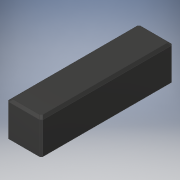
# Autodesk Inventor part: 1-Battery-Case
Saved by Autodesk Inventor 2019 (Build 230136000, 136)
## iProperties
Created: 2018-11-25
Part Number: 1-Battery-Case
Material: Generic
Document SubType Name: Modeling
Designer: lateSWE
Density: 1 g/cm^3
Appearance: Default
Author: lateSWE
Autodesk Inventor part; units mm, degrees
ref_plane "YZ Plane" through (0, 0, 0) normal (1, 0, 0) x (0, 1, 0)
ref_plane "XZ Plane" through (0, 0, 0) normal (0, 1, 0) x (-1, 0, 0)
ref_plane "XY Plane" through (0, 0, 0) normal (0, 0, 1) x (1, 0, 0)
sketch "Sketch1" plane through (0, 0, 0) normal (0, 0, 1) x (1, 0, 0)
  line L0 (0, 0) -> (22.5, 0)
  line L1 (22.5, 0) -> (22.5, 22.5)
  line L2 (22.5, 22.5) -> (0, 22.5)
  line L3 (0, 22.5) -> (0, 0)
  line L4 (0, 0) -> (20.5, 0)
  line L5 (20.5, 0) -> (20.5, 2)
  line L6 (20.5, 2) -> (0, 2)
  line L7 (0, 2) -> (0, 0)
  line L8 (22.5, 0) -> (20.5, 0)
  line L9 (20.5, 0) -> (20.5, 20.5)
  line L10 (20.5, 20.5) -> (22.5, 20.5)
  line L11 (22.5, 20.5) -> (22.5, 0)
  line L12 (22.5, 22.5) -> (2, 22.5)
  line L13 (2, 22.5) -> (2, 20.5)
  line L14 (2, 20.5) -> (22.5, 20.5)
  line L15 (22.5, 20.5) -> (22.5, 22.5)
  line L16 (0, 22.5) -> (2, 22.5)
  line L17 (2, 22.5) -> (2, 2)
  line L18 (2, 2) -> (0, 2)
  line L19 (0, 2) -> (0, 22.5)
  line L20 (2, 2) -> (20.5, 2)
  line L21 (20.5, 2) -> (20.5, 20.5)
  line L22 (20.5, 20.5) -> (2, 20.5)
  line L23 (2, 20.5) -> (2, 2)
  dimension "d0" = 22.5
  dimension "d1" = 22.5
  dimension "d2" = 20.5
  dimension "d3" = 2
  dimension "d4" = 2
  dimension "d5" = 20.5
  dimension "d6" = 20.5
  dimension "d7" = 2
  dimension "d8" = 2
  dimension "d9" = 20.5
  dimension "d10" = 18.5
  dimension "d11" = 18.5
  constraints: 48 end point, 12 parallel, 6 horizontal, 6 perpendicular
  measures "d0" distance of L2.end L1.end
  measures "d1" distance of L1.end L0.end
  measures "d2" distance of L6.end L5.end
  measures "d3" distance of L5.end L4.end
  measures "d4" distance of L9.end L10.end
  measures "d5" distance of L8.end L9.end
  measures "d6" distance of L14.end L13.end
  measures "d7" distance of L13.end L12.end
  measures "d8" distance of L17.end L18.end
  measures "d9" distance of L16.end L17.end
  measures "d10" distance of L22.end L9.end
  measures "d11" distance of L9.end L20.end
extrude "Extrusion1" add sketch "Sketch1" along normal blind 86.75
sketch "Sketch6" plane through (0, 0, 0) normal (0, -1, 0) x (1, 0, 0)
  line L0 (0, 0) -> (22.5, 0) projected
  line L1 (0, 0) -> (20.5, 0)
  line L2 (20.5, 0) -> (20.5, 2)
  line L3 (20.5, 2) -> (0, 2)
  line L4 (0, 2) -> (0, 0)
  line L5 (22.5, 0) -> (22.5, 86.75) projected
  line L6 (22.5, 0) -> (20.5, 0)
  line L7 (20.5, 0) -> (20.5, 84.75)
  line L8 (20.5, 84.75) -> (22.5, 84.75)
  line L9 (22.5, 84.75) -> (22.5, 0)
  line L10 (22.5, 86.75) -> (2, 86.75)
  line L11 (2, 86.75) -> (2, 84.75)
  line L12 (2, 84.75) -> (22.5, 84.75)
  line L13 (22.5, 84.75) -> (22.5, 86.75)
  line L14 (0, 0) -> (0, 86.75) projected
  line L15 (0, 86.75) -> (2, 86.75)
  line L16 (2, 86.75) -> (2, 2)
  line L17 (2, 2) -> (0, 2)
  line L18 (0, 2) -> (0, 86.75)
  line L19 (20.5, 84.75) -> (2, 84.75)
  line L20 (2, 84.75) -> (2, 2)
  line L21 (2, 2) -> (20.5, 2)
  line L22 (20.5, 2) -> (20.5, 84.75)
  dimension "d28" = 20.5
  dimension "d29" = 2
  dimension "d30" = 2
  dimension "d31" = 84.75
  dimension "d32" = 20.5
  dimension "d33" = 2
  dimension "d34" = 2
  dimension "d35" = 84.75
  dimension "d36" = 18.5
  dimension "d37" = 82.75
  constraints: 40 end point, 10 parallel, 5 horizontal, 5 perpendicular
  measures "d28" distance of L3.end L2.end
  measures "d29" distance of L2.end L1.end
  measures "d30" distance of L7.end L8.end
  measures "d31" distance of L6.end L7.end
  measures "d32" distance of L12.end L11.end
  measures "d33" distance of L11.end L10.end
  measures "d34" distance of L16.end L17.end
  measures "d35" distance of L15.end L16.end
  measures "d36" distance of L21.end L16.end
  measures "d37" distance of L16.end L19.end
extrude "Extrusion5" cut sketch "Sketch6" against normal blind 20.5 contours L3 L16 L12 L7
chamfer "Chamfer1" distance 1.5 angle 45 4 edges at (11.25, 22.5, 0) (22.5, 22.5, 43.375) (0, 22.5, 43.375) (11.25, 22.5, 86.75)
chamfer "Chamfer2" distance 1 angle 45 4 edges at (0, 10.5, 86.75) (22.5, 10.5, 86.75) (0, 10.5, 0) (22.5, 10.5, 0)
chamfer "Chamfer3" distance 0.8165 angle 45 4 edges at (1, 22, 85.75) (21.5, 22, 85.75) (21.5, 22, 1) (1, 22, 1)
body "Solid1"
